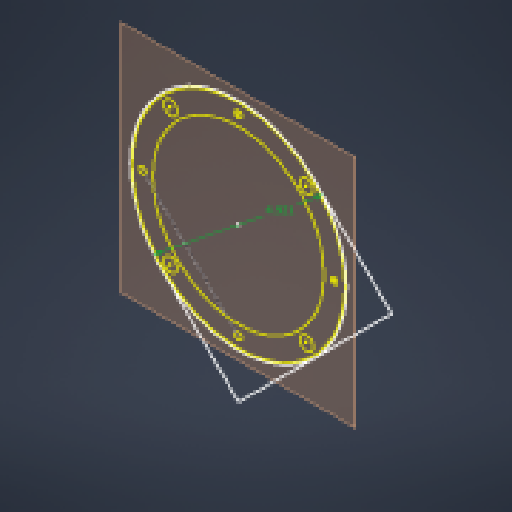
# Autodesk Inventor part: AxisBoard
Saved by Autodesk Inventor 2024 (Build 280153000, 153)
## iProperties
Created: 2023-10-21
Part Number: AxisBoard
Material: Generic
Document SubType Name: Modeling
Designer: range
Density: 1 g/cm^3
Appearance: Default
Author: range
Autodesk Inventor part; units mm, degrees
ref_plane "YZ Plane" through (0, 0, 0) normal (1, 0, 0) x (0, 1, 0)
ref_plane "XZ Plane" through (0, 0, 0) normal (0, 1, 0) x (-1, 0, 0)
ref_plane "XY Plane" through (0, 0, 0) normal (0, 0, 1) x (1, 0, 0)
ref_plane "Work Plane1" through (0, 0, 0) normal (0, 0, 1) x (1, 0, 0)
sketch "Sketch1" plane through (0, 0, 0) normal (0, 0, 1) x (1, 0, 0)
  circle A0 centre (0, 55.5) radius 2 projected
  circle A1 centre (55.5, 0) radius 2 projected
  circle A2 centre (-55.5, 0) radius 2 projected
  circle A3 centre (0, -55.5) radius 2 projected
  circle A4 centre (-39.2444, -39.2444) radius 4 projected
  circle A5 centre (39.2444, -39.2444) radius 4 projected
  circle A6 centre (-39.2444, 39.2444) radius 4 projected
  circle A7 centre (39.2444, 39.2444) radius 4 projected
  circle A8 centre (0, 0) radius 61.5 projected
  circle A9 centre (0, 0) radius 49.5 projected
  circle A10 centre (0, 0) radius 62.5
  line L0 (88.3883, 0) -> (0, -88.3883)
  line L1 (0, -55.5) -> (-55.5, 0) construction
  line L2 (88.3883, 0) -> (44.1942, 44.1942)
  line L3 (0, -88.3883) -> (-44.1942, -44.1942)
  point P0 (0, 0)
  dimension "d0" = 125
  constraints: 8 end point, 3 perpendicular, 3 tangent, 2 point on circle, 1 centre point, 1 coincident
  measures "d0" diameter of A10
extrude "Extrusion1" add sketch "Sketch1" along normal blind 6.35 contours A4 | A5 | A6 | A7 | A8 | A10 | A10 L2 L0 | L0 L3 A10
body "Solid1"
